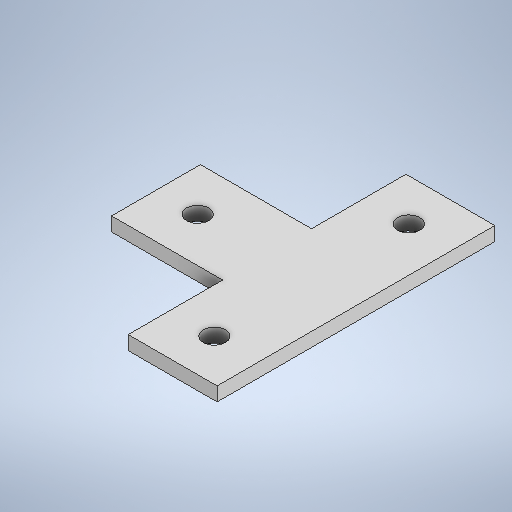
# Autodesk Inventor part: 2020T
Saved by Autodesk Inventor 2025.1 (Build 291241000, 241)
## iProperties
Created: 2025-12-01
Part Number: 2020T
Material: Generic
Document SubType Name: Modeling
Designer: Juxin
Density: 1 g/cm^3
Appearance: Default
Author: Juxin
Autodesk Inventor part; units mm, degrees
ref_plane "YZ Plane" through (0, 0, 0) normal (1, 0, 0) x (0, 1, 0)
ref_plane "XZ Plane" through (0, 0, 0) normal (0, 1, 0) x (-1, 0, 0)
ref_plane "XY Plane" through (0, 0, 0) normal (0, 0, 1) x (1, 0, 0)
sketch "Sketch1" plane through (0, 0, 0) normal (0, 1, 0) x (-1, 0, 0)
  line L0 (3.0436, 8.4522) -> (-17.2764, 8.4522)
  line L1 (-17.2764, 8.4522) -> (-17.2764, -55.0478)
  line L2 (-17.2764, -55.0478) -> (3.0436, -55.0478)
  line L3 (3.0436, -55.0478) -> (3.0436, 8.4522)
  line L4 (3.0436, -23.2978) -> (28.4436, -23.2978)
  line L5 (28.4436, -23.2978) -> (28.4436, -13.1378)
  line L6 (28.4436, -13.1378) -> (3.0436, -13.1378)
  line L7 (28.4436, -23.2978) -> (28.4436, -33.4578)
  line L8 (28.4436, -33.4578) -> (3.0436, -33.4578)
  line L9 (-7.1164, 8.4522) -> (-7.1164, -1.0728)
  line L10 (-7.1164, -55.0478) -> (-7.1164, -45.5228)
  circle A0 centre (-7.1164, -1.0728) radius 2.54
  circle A1 centre (-7.1164, -45.5228) radius 2.54
  line L11 (28.4436, -23.2978) -> (18.9186, -23.2978)
  circle A2 centre (18.9186, -23.2978) radius 2.54
  point P0 (0, 0)
  dimension "d0" = 20.32
  dimension "d1" = 63.5
  dimension "d2" = 25.4
  dimension "d3" = 10.16
  dimension "d4" = 10.16
  dimension "d5" = 9.525
  dimension "d6" = 9.525
  dimension "d7" = 5.08
  dimension "d8" = 5.08
  dimension "d9" = 9.525
  dimension "d10" = 5.08
  constraints: 24 end point, 4 perpendicular, 4 point on line, 3 centre point, 3 coincident, 3 midpoint, 2 horizontal, 2 parallel
  measures "d0" distance of L2.end L1.end
  measures "d1" distance of L1.end L0.end
  measures "d2" distance of L4.start L4.end
  measures "d3" distance of L4.end L5.end
  measures "d4" distance of L4.end L7.end
  measures "d5" distance of L9.start L9.end
  measures "d6" distance of L10.start L10.end
  measures "d7" diameter of A0
  measures "d8" diameter of A1
  measures "d9" distance of L4.end L11.end
  measures "d10" diameter of A2
extrude "Extrusion1" add sketch "Sketch1" along normal blind 3.175 contours L3 L2 L1 L0 | L6 L5 L4 A2 L3 | L4 A2 L7 L8 L3
body "Solid1"
